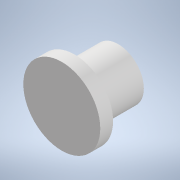
# Autodesk Inventor part: glide lejre bushing
Saved by Autodesk Inventor 2022.2 (Build 262287010, 287A)
## iProperties
Created: 2022-04-19
Part Number: glide lejre bushing
Material: Brass, Soft Yellow
Document SubType Name: Modeling
Designer: Finn Oriwohl
Density: 8.47 g/cm^3
Appearance: Brass - Satin
Author: Finn Oriwohl
Autodesk Inventor part; units mm, degrees
ref_plane "YZ Plane" through (0, 0, 0) normal (1, 0, 0) x (0, 1, 0)
ref_plane "XZ Plane" through (0, 0, 0) normal (0, 1, 0) x (-1, 0, 0)
ref_plane "XY Plane" through (0, 0, 0) normal (0, 0, 1) x (1, 0, 0)
sketch "Sketch1" plane through (0, 0, 0) normal (0, 0, 1) x (1, 0, 0)
  circle A0 centre (0, 1.5) radius 10 projected
  circle A1 centre (0, 1.5) radius 10 projected
  circle A2 centre (0, 1.5) radius 15
  circle A3 centre (0, 1.5) radius 7.5
  point P0 (0, 0)
  dimension "d0" = 30
  dimension "d1" = 15
  constraints: 2 centre point, 2 coincident
  measures "d0" diameter of A2
  measures "d1" diameter of A3
ref_plane "Work Plane1" through (-46.5047, -36.7959, -17) normal (0, 0, -1) x (0, 1, 0)
extrude "Extrusion1" add sketch "Sketch1" against normal up to surface (17 mm away) contours A0
sketch "Sketch2" plane through (0, 1.5, 0) normal (0, 0, 1) x (1, 0, 0)
  circle A0 centre (0, 0) radius 10 projected
  circle A1 centre (0, 0) radius 7.5 projected
  circle A2 centre (0, 0) radius 15
  point P0 (0, -1.5)
  dimension "d4" = 30
  constraints: 1 centre point, 1 coincident
  measures "d4" diameter of A2
extrude "Extrusion2" add sketch "Sketch2" along normal blind 5 contours A0 | A1 | A2
body "Solid1"
